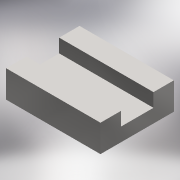
# Autodesk Inventor part: MGN12C
Saved by Autodesk Inventor 2021 (Build 250183000, 183)
## iProperties
Created: 2020-05-08
Part Number: MGN12C
Material: Stainless Steel
Document SubType Name: Modeling
Designer: Remo
Density: 8 g/cm^3
Appearance: Semi-Polished
Mass: 56.9212 g
Surface Area: 36.0989 cm^2
Volume: 7.11516 cm^3
Description: HIWIN MGN12C Linear Bearing Block
Author: Remo
Autodesk Inventor part; units mm, degrees
ref_plane "YZ Plane" through (0, 0, 0) normal (1, 0, 0) x (0, 1, 0)
ref_plane "XZ Plane" through (0, 0, 0) normal (0, 1, 0) x (-1, 0, 0)
ref_plane "XY Plane" through (0, 0, 0) normal (0, 0, 1) x (1, 0, 0)
sketch "Sketch1" plane through (0, 0, 0) normal (0, 0, 1) x (1, 0, 0)
  line L0 (17.35, -13.5) -> (-17.35, -13.5)
  line L1 (-17.35, -13.5) -> (-17.35, 13.5)
  line L2 (-17.35, 13.5) -> (17.35, 13.5)
  line L3 (17.35, 13.5) -> (17.35, -13.5)
  line L4 (17.35, -13.5) -> (-17.35, 13.5) construction
  line L5 (-17.35, -13.5) -> (17.35, 13.5) construction
  point P0 (0, 0)
  dimension "d0" = 27
  dimension "d1" = 34.7
  constraints: 12 end point, 2 midpoint, 2 parallel, 1 horizontal, 1 perpendicular
  measures "d0" distance of L2.end L0.start
  measures "d1" distance of L0.start L0.end
extrude "Extrusion1" add sketch "Sketch1" along normal blind 10
sketch "Sketch2" plane through (0, 0, 10) normal (0, 0, 1) x (1, 0, 0)
  line L0 (17.35, -6) -> (-17.35, -6)
  line L1 (-17.35, -6) -> (-17.35, 6)
  line L2 (-17.35, 6) -> (17.35, 6)
  line L3 (17.35, 6) -> (17.35, -6)
  line L4 (17.35, -6) -> (-17.35, 6) construction
  line L5 (-17.35, -6) -> (17.35, 6) construction
  point P0 (0, 0)
  point P1 (17.35, 13.5)
  dimension "d4" = 12
  constraints: 12 end point, 2 midpoint, 2 parallel, 1 horizontal, 1 perpendicular, 1 vertical alignment
  measures "d4" distance between parallel lines of L0 L2
extrude "Extrusion2" cut sketch "Sketch2" against normal blind 5
sketch "Sketch3" plane through (0, 0, 0) normal (0, 0, -1) x (-1, 0, 0)
  point P0 (0, 0)
  point P1 (-7.5, 10)
  point P2 (-7.5, -10)
  point P3 (7.5, 10)
  point P4 (7.5, -10)
  dimension "d7" = 20
  dimension "d8" = 10
  dimension "d9" = 15
  dimension "d10" = 7.5
  constraints: 2 horizontal alignment, 2 vertical alignment
  measures "d7" distance of point (-7.5, -10) point (-7.5, 10)
  measures "d8" vertical distance of point (-7.5, 10) point (0, 0)
  measures "d9" distance of point (7.5, 10) point (-7.5, 10)
  measures "d10" horizontal distance of point (0, 0) point (-7.5, 10)
hole "Hole1" at (7.5, 10, 0) at (7.5, -10, 0) at (-7.5, 10, 0) at (-7.5, -10, 0) direction (0, 0, 1) diameter 2.459 depth 8.8 tip angle 118 thread size "M3x0.5" class "6H" standard "ISO Metric profile"
equation "\"d8\" = 0.5 * d7"
equation "\"d10\" = 0.5 * d9"
body "Solid1"
